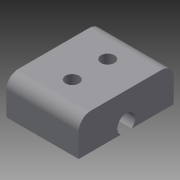
# Autodesk Inventor part: axle holder
Saved by Autodesk Inventor 2015 (Build 190159000, 159)
## iProperties
Created: 2014-10-03
Part Number: axle holder
Material: Generic
Document SubType Name: Modeling
Designer: jesse
Density: 1 g/cm^3
Appearance: Default
Author: jesse
Autodesk Inventor part; units mm, degrees
ref_plane "YZ Plane" through (0, 0, 0) normal (1, 0, 0) x (0, 1, 0)
ref_plane "XZ Plane" through (0, 0, 0) normal (0, 1, 0) x (-1, 0, 0)
ref_plane "XY Plane" through (0, 0, 0) normal (0, 0, 1) x (1, 0, 0)
sketch "Sketch1" plane through (0, 0, 0) normal (1, 0, 0) x (0, 1, 0)
  arc A0 (-1.8542, -1.4222) -> (-1.8542, 1.4222) centre (0, 0) ccw
  line L0 (-2.4782, 12.4968) -> (4.3758, 12.4968)
  line L1 (7.5508, 9.3218) -> (7.5508, -9.3218)
  line L2 (4.3758, -12.4968) -> (-1.8542, -12.4968)
  line L3 (-1.8542, 12.4968) -> (-2.4782, 12.4968)
  line L4 (2.3368, 0) -> (2.3368, -12.4968) construction
  line L5 (0, 0) -> (3.6666, 0) construction
  line L6 (3.6666, 0) -> (3.6666, 12.4968) construction
  line L7 (3.6666, 0) -> (3.6666, -12.4968) construction
  arc A1 (7.5508, 9.3218) -> (4.3758, 12.4968) centre (4.3758, 9.3218) ccw
  arc A2 (4.3758, -12.4968) -> (7.5508, -9.3218) centre (4.3758, -9.3218) ccw
  line L8 (-1.8542, -12.4968) -> (-1.8542, -1.4222)
  line L9 (-1.8542, 1.4222) -> (-1.8542, 12.4968)
  dimension "d0" = 4.6736
  dimension "d4" = 10.16
  dimension "d5" = 3.175
  constraints: 20 end point, 8 perpendicular, 7 point on circle, 5 point on line, 5 tangent, 3 centre point, 2 horizontal, 1 coincident, 1 collinear, 1 equal radius
  measures "d0" diameter of A0
  measures "d4" distance edge to line of A0 L2
  measures "d5" radius of A1
extrude "Extrusion1" add sketch "Sketch1" along normal blind 19.05
sketch "Sketch2" plane through (0, 7.5508, 9.3218) normal (0, 1, 0) x (1, 0, 0)
  line L0 (0, 18.6436) -> (0, 0) construction
  line L1 (0, 0) -> (19.05, 0) construction
  line L2 (19.05, 18.6436) -> (19.05, 0) construction
  line L3 (0, 18.6436) -> (19.05, 18.6436) construction
  line L4 (0, 9.3218) -> (19.05, 9.3218) construction
  line L5 (9.525, 9.3218) -> (9.525, 18.6436) construction
  line L6 (0, 18.6436) -> (19.05, 18.6436) construction
  line L7 (9.525, 9.3218) -> (9.525, 0) construction
  line L8 (0, 0) -> (19.05, 0) construction
  circle A0 centre (9.525, 13.9827) radius 1.778
  circle A1 centre (9.525, 4.6609) radius 1.778
  dimension "d8" = 3.556
  constraints: 6 end point, 6 midpoint, 2 centre point, 1 equal radius
  measures "d8" diameter of A0
extrude "Extrusion2" cut sketch "Sketch2" against normal blind 19.05
body "Solid1"
